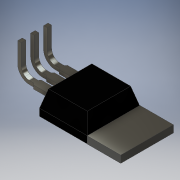
# Autodesk Inventor part: TO-220_UnderHeat
Saved by Autodesk Inventor 2016 (Build 200138000, 138)
## iProperties
Created: 2016-09-10
Part Number: TO-220_UnderHeat
Material: Generic
Document SubType Name: Modeling
Designer: jfixelle
Density: 1 g/cm^3
Appearance: Black
Author: jfixelle
Autodesk Inventor part; units mm, degrees
ref_plane "YZ Plane" through (0, 0, 0) normal (1, 0, 0) x (0, 1, 0)
ref_plane "XZ Plane" through (0, 0, 0) normal (0, 1, 0) x (-1, 0, 0)
sketch "Sketch1" plane through (0, 0, 0) normal (0, 1, 0) x (-1, 0, 0)
  line L0 (4.7, 5.15) -> (-4.7, 5.15)
  line L1 (-4.7, 5.15) -> (-4.7, -5.15)
  line L2 (-4.7, -5.15) -> (4.7, -5.15)
  line L3 (4.7, -5.15) -> (4.7, 5.15)
  point P0 (0, 0)
  dimension "d0" = 9.4
  dimension "d1" = 4.7
  dimension "d2" = 10.3
  dimension "d3" = 5.15
  constraints: 8 end point, 2 parallel, 1 horizontal, 1 perpendicular
  measures "d0" distance of L1.end L2.end
  measures "d1" distance from line of point (0, 0) L3
  measures "d2" distance of L0.end L1.end
  measures "d3" distance from line of L2 point (0, 0)
extrude "Extrusion1" add sketch "Sketch1" along normal blind 4.7
chamfer "Chamfer1" distance 3.3 angle 15 1 edges at (0, 4.7, 5.15) measured on face at (-1.5667, 1.5667, 5.15)
chamfer "Chamfer2" distance 3.3 angle 15 1 edges at (4.7, 4.7, -0.4421) measured on face at (4.7, 3.1333, -2.0114)
chamfer "Chamfer3" distance 3.3 angle 15 1 edges at (-0.4421, 4.7, -5.15) measured on face at (-1.8614, 3.1333, -5.15)
chamfer "Chamfer4" distance 3.3 angle 15 1 edges at (-4.7, 4.7, 0) measured on face at (-4.7, 2.5, -1.4219)
sketch "Sketch2" plane through (0, 0, 0) normal (0, -1, 0) x (1, 0, 0)
  line L0 (4.7, 5.15) -> (4.7, -5.15) projected
  line L1 (11.3, -5.15) -> (11.3, 5.1662)
  line L2 (11.3, 5.1662) -> (4.7, 5.1662)
  line L3 (4.7, 5.1662) -> (4.7, -5.15)
  line L4 (-4.7, 5.15) -> (4.7, 5.15) projected
  line L5 (11.3, -5.15) -> (11.3, -5.1902)
  line L6 (11.3, -5.1902) -> (4.7, -5.1902)
  line L7 (4.7, -5.1902) -> (4.7, -5.15)
  point P0 (0, 0)
  dimension "d18" = 6.6
  constraints: 12 end point, 2 perpendicular, 1 parallel, 1 vertical
  measures "d18" distance of L0.end L1.start
extrude "Extrusion2" add sketch "Sketch2" against normal blind 1.4 and the other way blind 0.01
ref_plane "Work Plane1" through (0, 2.6, 0) normal (0, -1, 0) x (1, 0, 0)
sketch "Sketch3" plane through (0, 2.6, 0) normal (0, -1, 0) x (1, 0, 0)
  line L0 (-4.304, -0.8) -> (-8, -0.8)
  line L1 (-8, -0.8) -> (-8, 0.8)
  line L2 (-8, 0.8) -> (-4.304, 0.8)
  line L3 (-4.304, 0.8) -> (-4.304, -0.8)
  line L4 (-4.7, -5.15) -> (-4.7, 5.15) projected
  line L5 (-4.7, -5.15) -> (-4.7, 5.15) projected
  line L6 (-4.7, 0) -> (-3.1889, 0)
  line L7 (-8, -0.45) -> (-7.7, -0.8)
  line L8 (-8, 0.45) -> (-7.7, 0.8)
  point P0 (0, 0)
  dimension "d25" = 3.3
  dimension "d26" = 1.6
  dimension "d27" = 0.8
  dimension "d28" = 3
  dimension "d29" = 3
  dimension "d30" = 0.9
  dimension "d31" = 0.45
  constraints: 14 end point, 4 point on line, 2 horizontal, 2 parallel, 1 midpoint, 1 perpendicular
  measures "d25" distance between parallel lines of L1 L4
  measures "d26" distance of L0.end L1.end
  measures "d27" distance between parallel lines of L0 L6
  measures "d28" distance from line of L4 L7.end
  measures "d29" distance from line of L4 L8.end
  measures "d30" distance of L8.start L7.start
  measures "d31" distance from line of L6 L8.start
extrude "Extrusion3" add sketch "Sketch3" along normal mid plane 0.7 contours L7 L1 L8 L2 L4 L0 | L4 L6 L3 L0 | L4 L2 L3 L6
sketch "Sketch4" plane through (-8, 2.25, -0.45) normal (-1, 0, 0) x (0, 0, 1)
  line L0 (1.25, 0.7) -> (-0.35, 0.7) projected
  line L1 (1.25, 0) -> (-0.35, 0) projected
  line L2 (0.9, 0.7) -> (0, 0.7)
  line L3 (0, 0.7) -> (0, 0)
  line L4 (0, 0) -> (0.9, 0)
  line L5 (0.9, 0) -> (0.9, 0.7)
  line L6 (0.9, 0.7) -> (0.9, 0) projected
  line L7 (0.9, 0.126) -> (0.9, 0.1378)
  point P0 (0.45, -2.25)
  dimension "d34" = 0.9
  dimension "d35" = 0
  constraints: 10 end point, 4 point on line, 2 parallel, 1 horizontal, 1 perpendicular
  measures "d34" distance between parallel lines of L5 L3
  measures "d35" distance between parallel lines of L5 L6
sketch "Sketch5" plane through (0, 0, 0) normal (0, 0, 1) x (1, 0, 0)
  line L0 (-8, 2.95) -> (-8, 2.25) projected
  line L1 (-8, 2.6) -> (-8.8, 2.6)
  line L2 (-10.8, 4.6) -> (-10.8, 8.6)
  line L3 (-4.557, 8.6) -> (-13.8977, 8.6)
  line L4 (4.7, 0) -> (-4.7, 0) projected
  arc A0 (-10.8, 4.6) -> (-8.8, 2.6) centre (-8.8, 4.6) ccw
  point P0 (0, 0)
  dimension "d36" = 8.6
  dimension "d38" = 2.8
  dimension "d39" = 2
  constraints: 6 end point, 2 horizontal, 2 point on circle, 2 tangent, 1 centre point, 1 midpoint, 1 perpendicular, 1 point on line
  measures "d36" distance between parallel lines of L4 L3
  measures "d38" distance between parallel lines of L2 L0
  measures "d39" radius of A0
sweep "Sweep1" add profiles "Sketch4" path "Sketch5" path curves L1 A0 L2
pattern_linear "Rectangular Pattern1" count 3 spacing 2.54 along (0, 0, -1) of "Extrusion3", "Sweep1" first direction both ways yes
body "Solid1"
